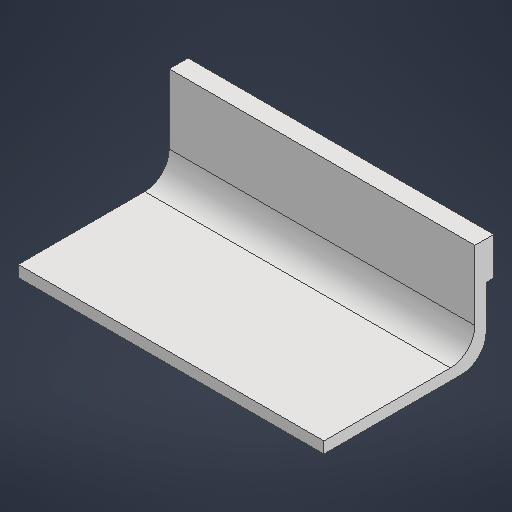
# Autodesk Inventor part: 前舵机位置控制
Saved by Autodesk Inventor 2025 (Build 290162000, 162)
## iProperties
Created: 2025-12-02
Part Number: 前舵机位置控制
Material: 常规
Document SubType Name: Modeling
Designer: HZD
Density: 1 g/cm^3
Appearance: 默认
Author: HZD
Autodesk Inventor part; units mm, degrees
ref_plane "YZ Plane" through (0, 0, 0) normal (1, 0, 0) x (0, 1, 0)
ref_plane "XZ Plane" through (0, 0, 0) normal (0, 1, 0) x (-1, 0, 0)
ref_plane "XY Plane" through (0, 0, 0) normal (0, 0, 1) x (1, 0, 0)
sketch "草图2" plane through (0, 0, 0) normal (0, 1, 0) x (-1, 0, 0)
  line L0 (-73.613, -25.5176) -> (7.387, -25.5176) projected
  line L1 (-73.613, -25.5176) -> (-73.613, 14.4824) projected
  line L2 (7.387, 14.4824) -> (-73.613, 14.4824) projected
  line L3 (7.387, -25.5176) -> (7.387, 14.4824) projected
  point P0 (0, 0)
extrude "拉伸1" add sketch "草图2" along normal blind 3
sketch "草图3" plane through (-7.387, 0, -25.5176) normal (-1, 0, 0) x (0, 0, 1)
  line L0 (0, 0) -> (40, 0) projected
  line L1 (0, 0) -> (-3, 0)
  line L2 (-3, 0) -> (-3, 26)
  line L3 (-3, 26) -> (0, 26)
  line L4 (0, 26) -> (0, 0)
  point P0 (25.5176, 0)
  dimension "d2" = 3
  dimension "d3" = 26
  constraints: 8 end point, 2 parallel, 1 horizontal, 1 perpendicular
  measures "d2" distance of L2.end L3.end
  measures "d3" distance between parallel lines of L1 L3
extrude "拉伸2" add sketch "草图3" against normal up to surface (81 mm away)
fillet "圆角1" radius 6.5 2 edges at (33.113, 3, -25.5176) (33.113, 0, -28.5176)
sketch "草图4" plane through (73.613, 26, -28.5176) normal (0, 0, -1) x (-1, 0, 0)
  line L0 (3, -1.1) -> (78, -1.1) projected
  line L1 (3, -76.1) -> (3, -1.1) projected
  line L2 (78, -76.1) -> (3, -76.1) projected
  line L3 (78, -1.1) -> (78, -76.1) projected
  line L4 (81, -79.1) -> (0, -79.1)
  line L5 (0, -79.1) -> (0, 1.9)
  line L6 (0, 1.9) -> (81, 1.9)
  line L7 (81, 1.9) -> (81, -79.1)
  line L8 (81, -8.1) -> (0, -8.1)
  line L9 (71, 1.9) -> (71, -79.1)
  line L10 (37.5, -29.6254) -> (37.5, -58.9595)
  line L11 (4, 1.9) -> (4, -79.1)
  point P0 (73.613, -26)
  point P1 (3, -8.1)
  point P2 (78, -8.1)
  dimension "d8" = 3
  dimension "d9" = 10
  dimension "d10" = 10
  constraints: 16 end point, 4 point on line, 2 perpendicular, 2 symmetric about line, 1 vertical, 3 other
  measures "d8" distance between parallel lines of L3 L7
  measures "d9" distance between parallel lines of L6 L8
  measures "d10" distance between parallel lines of L7 L9
extrude "拉伸3" add sketch "草图4" along normal blind 2 contours L1 L8 L5 L6 L11 L0 | L11 L6 L9 L0 | L9 L6 L7 L8 L3 L0
sketch "草图5" plane through (73.613, 26, -28.5176) normal (0, 0, 1) x (1, 0, 0)
  line L0 (0, 1.9) -> (0, 0) projected
  line L1 (-81, 1.9) -> (0, 1.9) projected
  line L2 (-81, 0) -> (-81, 1.9) projected
  line L3 (-81, 0) -> (0, 0) projected
  point P0 (-73.613, -26)
extrude "拉伸4" add sketch "草图5" along normal up to surface (3 mm away)
sketch "草图6" plane through (0, 0, 0) normal (0, -1, 0) x (1, 0, 0)
  point P0 (0, 0)
sketch "草图7" plane through (0, 0, 0) normal (0, -1, 0) x (1, 0, 0)
  line L0 (-4.387, -23.5176) -> (-7.387, -23.5176) projected
  line L1 (-4.387, -23.5176) -> (-4.387, 10.4824) projected
  line L2 (-4.387, 10.4824) -> (70.613, 10.4824) projected
  line L3 (70.613, 10.4824) -> (70.613, -23.5176) projected
  line L4 (73.613, -23.5176) -> (70.613, -23.5176) projected
  line L5 (73.613, -23.5176) -> (73.613, 14.4824) projected
  line L6 (-7.387, 14.4824) -> (73.613, 14.4824) projected
  line L7 (-7.387, -23.5176) -> (-7.387, 14.4824) projected
  circle A0 centre (-2.387, 7.4824) radius 0.8
  circle A1 centre (-2.387, 4.9824) radius 0.8
  circle A2 centre (-2.387, 2.4824) radius 0.8
  line L8 (-1.137, 10.1034) -> (-1.137, 2.8167)
  circle A3 centre (0.113, 7.4824) radius 0.8
  circle A4 centre (0.113, 4.9824) radius 0.8
  circle A5 centre (0.113, 2.4824) radius 0.8
  point P0 (0, 0)
  dimension "d16" = 2.5
  dimension "d17" = 2.5
  dimension "d18" = 1.6
  dimension "d19" = 1.6
  dimension "d20" = 1.6
  dimension "d21" = 2
  dimension "d22" = 1.25
  dimension "d32" = 3
  constraints: 6 centre point, 3 symmetric about line, 2 end point, 2 vertical alignment, 1 vertical, 3 other
  measures "d16" distance of A1.centre A0.centre
  measures "d17" distance of A1.centre A2.centre
  measures "d18" diameter of A2
  measures "d19" diameter of A1
  measures "d20" diameter of A0
  measures "d21" distance from line of A1.centre L1
  measures "d22" distance from line of A1.centre L8
  measures "d32" distance from line of L2 A3.centre
extrude "拉伸5" cut sketch "草图7" against normal blind 2 contours A0 | A1 | A2 | A3 | A4 | A5
fillet "圆角3" radius 0.3 6 edges at (-3.187, 2, 7.4824) (-0.687, 2, 7.4824) (-0.687, 2, 4.9824) (-3.187, 2, 4.9824) (-0.687, 2, 2.4824) (-3.187, 2, 2.4824)
chamfer "倒角1" distance 0.5 angle 45 6 edges at (-0.687, 0, 7.4824) (-0.687, 0, 4.9824) (-0.687, 0, 2.4824) (-3.187, 0, 4.9824) (-3.187, 0, 7.4824) (-3.187, 0, 2.4824)
pattern_linear "矩形阵列1" count 10 spacing 7.6 along (1, 0, 0) of "拉伸5", "圆角3", "倒角1"
